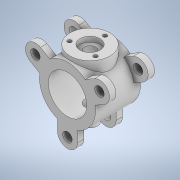
# Autodesk Inventor part: Corpo da Valvula
Saved by Autodesk Inventor 2020 (Build 240168000, 168)
## iProperties
Created: 2022-04-26
Part Number: Corpo da Valvula
Material: Genérico
Document SubType Name: Modeling
Designer: robofei
Density: 1 g/cm^3
Appearance: Padrão
Author: robofei
Autodesk Inventor part; units mm, degrees
ref_plane "YZ Plane" through (0, 0, 0) normal (1, 0, 0) x (0, 1, 0)
sketch "Esboço1" plane through (0, 0, 0) normal (0, 0, 1) x (1, 0, 0)
  circle A0 centre (0, 0) radius 140
  circle A1 centre (0, 0) radius 96
  dimension "d0" = 280
  dimension "d1" = 192
  constraints: 2 centre point, 2 coincident
  measures "d0" diameter of A0
  measures "d1" diameter of A1
extrude "Extrusão1" add sketch "Esboço1" along normal mid plane 225
ref_plane "Plano de trabalho1" through (0, 160, 0) normal (0, 1, 0) x (-1, 0, 0)
sketch "Esboço2" plane through (0, 160, 0) normal (0, 1, 0) x (-1, 0, 0)
  circle A0 centre (0, 0) radius 100
  dimension "d5" = 200
  constraints: 1 centre point, 1 coincident
  measures "d5" diameter of A0
extrude "Extrusão2" add sketch "Esboço2" against normal up to next
ref_plane "Plano de trabalho2" through (0, -175, 0) normal (0, 1, 0) x (-1, 0, 0)
sketch "Esboço3" plane through (0, -175, 0) normal (0, 1, 0) x (-1, 0, 0)
  circle A0 centre (0, 0) radius 37.5
  dimension "d9" = 75
  constraints: 1 centre point, 1 coincident
  measures "d9" diameter of A0
extrude "Extrusão3" add sketch "Esboço3" along normal up to next
sketch "Esboço4" plane through (0, 160, 0) normal (0, 1, 0) x (1, 0, 0)
  circle A0 centre (0, 0) radius 50
  dimension "d12" = 100
  constraints: 1 centre point, 1 coincident
  measures "d12" diameter of A0
extrude "Extrusão4" cut sketch "Esboço4" against normal blind 25
sketch "Esboço5" plane through (0, 135, 0) normal (0, 1, 0) x (1, 0, 0)
  circle A0 centre (0, 0) radius 28
  dimension "d15" = 56
  constraints: 1 centre point, 1 coincident
  measures "d15" diameter of A0
extrude "Extrusão5" cut sketch "Esboço5" against normal blind 285
sketch "Esboço6" plane through (0, 160, 0) normal (0, 1, 0) x (1, 0, 0)
  circle A0 centre (0, 75) radius 10
  circle A1 centre (-64.9519, -37.5) radius 10
  circle A2 centre (64.9519, -37.5) radius 10
  point P0 (0, 0)
  dimension "d18" = 20
  dimension "d19" = 75
  dimension "d22" = 360
  constraints: 3 centre point, 7 other
  measures "d18" diameter of A0
  measures "d19" distance of point (0, 0) A0.centre
extrude "Extrusão6" cut sketch "Esboço6" against normal blind 15
sketch "Esboço7" plane through (0, 0, 112.5) normal (0, 0, 1) x (1, 0, 0)
  arc A0 (-50, -185) -> (50, -185) centre (0, -185) ccw
  circle A1 centre (0, -185) radius 23.5
  line L0 (50, -185) -> (50, -106.8082)
  line L1 (-50, -185) -> (-50, -106.8082)
  line L2 (50, -106.8082) -> (-50, -106.8082)
  point P0 (0, 0)
  dimension "d26" = 100
  dimension "d27" = 47
  dimension "d28" = 185
  constraints: 6 end point, 2 centre point, 2 point on circle, 2 tangent, 1 coincident, 1 horizontal, 1 vertical
  measures "d26" diameter of A0
  measures "d27" diameter of A1
  measures "d28" distance of A0.centre point (0, 0)
extrude "Extrusão7" add sketch "Esboço7" against normal blind 32
pattern_circular "Padrão circular1" count 3 over 360 about axis through (0, 0, 0) along (0, 0, 1) of "Extrusão7"
mirror "Espelhamento1" about plane through (0, 0, 0) normal (0, 0, 1) of "Extrusão7", "Padrão circular1"
